Autodesk Fusion 360 part; units mm, degrees
note: some values were not read from the file. Set by a fixed rule: which face or edge a step refers to.
(part 4 of 5)
sketch "Sketch4" plane through (0, 0, 0) normal (1, 0, 0) x (0, 0, -1)
  circle A0 centre (-14.7805, 3.85) radius 2.25 construction
  line L0 (-20.7805, 0) -> (-8.7805, 0) construction
  line L1 (-8.7805, 0) -> (-8.7805, 7.7) construction
  line L2 (-8.7805, 7.7) -> (-20.7805, 7.7) construction
  line L3 (-20.7805, 7.7) -> (-20.7805, 0) construction
  line L4 (8.7805, 0) -> (-8.7805, 0) construction
  line L5 (-8.7805, 0) -> (-8.7805, 7.7) construction
  line L6 (8.7805, 7.7) -> (-8.7805, 7.7) construction
  line L7 (-8.7805, 7.7) -> (-8.7805, 0) construction
  circle A1 centre (-14.7805, 3.85) radius 2.25 construction
  line L8 (-8.7805, 0) -> (-25.7687, 0) construction
  line L9 (-25.7687, 0) -> (-25.7687, 7.7) construction
  line L10 (-25.7687, 7.7) -> (-8.7805, 7.7) construction
  line L11 (-8.7805, 7.7) -> (-8.7805, 0) construction
  line L12 (8.7805, 0) -> (-23.2746, 0)
  line L13 (-23.2746, 0) -> (-23.2746, 7.7)
  line L14 (-23.2746, 7.7) -> (8.7805, 7.7)
  line L15 (8.7805, 7.7) -> (8.7805, 0)
  line L16 (-25.7687, 7.7) -> (-20.7805, 7.7) construction
  line L17 (8.7805, 7.7) -> (8.7805, 0)
  line L18 (8.7805, 0) -> (-8.7805, 0)
  line L19 (8.7805, 0) -> (8.7805, 7.7)
  line L20 (8.7805, 7.7) -> (-8.7805, 7.7)
  circle A2 centre (14.7805, 3.85) radius 2.25
  line L21 (8.7805, 0) -> (20.7805, 0)
  line L22 (20.7805, 0) -> (20.7805, 7.7)
  line L23 (20.7805, 7.7) -> (8.7805, 7.7)
  line L24 (8.7805, 7.7) -> (8.7805, 0)
  constraint horizontal L12
  constraint vertical L13
  constraint horizontal L14
  constraint vertical L15
  constraint coincident L10 L13.end
  constraint coincident L4.start L12.start
  constraint coincident L9.end L10.start
  constraint coincident L2.end L3.start
  constraint midpoint L13.end L16
extrude "Extrude4" cut sketch "Sketch4" against normal blind 9.755
ref_plane "WorkPlane1" through (9.4113, 3.85, 28.5317) normal (-0.487666, 0, 0.87303) x (0.87303, 0, 0.487666)
sketch "Sketch5" plane through (-9.9091, 0, 17.7395) normal (-0.487666, 0, 0.87303) x (0.87303, 0, 0.487666)
  line L0 (7.6399, 0) -> (7.6399, 7.7)
  line L1 (7.6399, 7.7) -> (11.3502, 7.7)
  line L2 (11.3502, 7.7) -> (11.3502, 0)
  line L3 (11.3502, 0) -> (7.6399, 0)
  circle A0 centre (21.8443, 3.85) radius 2.25
  line L4 (35.4044, 0) -> (13.8443, 0)
  line L5 (13.8443, 0) -> (13.8443, 7.7)
  line L6 (13.8443, 7.7) -> (35.4044, 7.7)
  line L7 (35.4044, 7.7) -> (35.4044, 0)
  line L8 (7.6399, 7.7) -> (27.1402, 7.7)
  line L9 (27.1402, 7.7) -> (27.1402, 0)
  line L10 (27.1402, 0) -> (7.6399, 0)
  line L11 (7.6399, 0) -> (7.6399, 7.7)
  line L12 (21.8443, 3.85) -> (21.8443, 7.7) construction
  line L13 (21.8443, 7.7) -> (35.4044, 7.7) construction
  point P0 (27.1402, 8)
  dimension "d37" = 15.79
  constraint horizontal L8
  constraint vertical L9
  constraint horizontal L10
  constraint vertical L11
  constraint coincident L4 L9.end
  constraint coincident L0.end L1.start
  constraint coincident A0.centre L12.start
  constraint coincident L6 L12.end
  constraint vertical L12
  constraint coincident L6.end L7.start
  constraint coincident L9 P0
  measures "d37" distance of L2 L9
extrude "Extrude5" cut sketch "Sketch5" along normal up to surface (4.25 mm away) contours L0 L1 L2 L3 L8 L10 L11 | L2 L5 L8 L10 | L4 L5 L6 L8 L9 L10
sketch "Sketch6" plane through (-11.9817, 0, 21.4499) normal (-0.487666, 0, 0.87303) x (0.87303, 0, 0.487666)
  line L0 (27.1402, 7.7) -> (27.1402, 0)
  line L1 (27.1402, 0) -> (35.4044, 0)
  line L2 (35.4044, 0) -> (35.4044, 7.7)
  line L3 (35.4044, 7.7) -> (27.1402, 7.7)
  line L4 (39.6544, 0) -> (35.4044, 0)
  line L5 (35.4044, 0) -> (35.4044, 7.7)
  line L6 (39.6544, 7.7) -> (35.4044, 7.7)
  line L7 (27.1402, 7.7) -> (39.6544, 7.7)
  line L8 (39.6544, 7.7) -> (39.6544, 0)
  line L9 (39.6544, 0) -> (27.1402, 0)
  line L10 (27.1402, 0) -> (27.1402, 7.7)
  line L11 (35.4044, 7.7) -> (35.4044, 0)
  constraint horizontal L7
  constraint vertical L8
  constraint horizontal L9
  constraint vertical L10
  constraint coincident L4.start L8.end
  constraint coincident L0.start L3.end
extrude "Extrude6" cut sketch "Sketch6" against normal up to surface (8.5 mm away)
equation "d19 = d4"
equation "d20 = ( -d22 / 2 mm ) * 1 mm"
equation "d22 = d1 + 6 mm"
equation "d31 = d32"

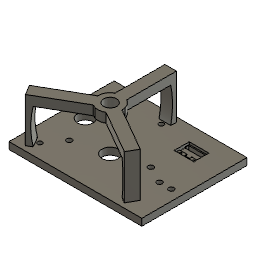
design "Strain Gauge Mount"
Autodesk Fusion 360 part; units mm, degrees
sketch "Sketch1" plane through (0, 0, 0) normal (0, 1, 0) x (1, 0, 0)
  line L0 (-47.5333, 52) -> (47.5333, 52) construction
  line L1 (47.5333, 52) -> (47.5333, -25) construction
  line L2 (47.5333, -25) -> (-47.5333, -25) construction
  line L3 (-47.5333, -25) -> (-47.5333, 52) construction
  line L4 (0, 8) -> (-6.9282, -4) construction
  line L5 (-6.9282, -4) -> (6.9282, -4) construction
  line L6 (6.9282, -4) -> (0, 8) construction
  line L7 (-2.5, 4.3301) -> (2.5, -4.3301) construction
  line L8 (2.5, -4.3301) -> (-42.5333, -30.3301) construction
  line L9 (-42.5333, -30.3301) -> (-47.5333, -21.6699) construction
  line L10 (-47.5333, -21.6699) -> (-2.5, 4.3301) construction
  line L11 (2.5, 4.3301) -> (-2.5, -4.3301) construction
  line L12 (-2.5, -4.3301) -> (42.5333, -30.3301) construction
  line L13 (42.5333, -30.3301) -> (47.5333, -21.6699) construction
  line L14 (2.5, 4.3301) -> (47.5333, -21.6699) construction
  line L15 (-5, 0) -> (-5, 52) construction
  line L16 (-5, 52) -> (5, 52) construction
  line L17 (5, 52) -> (5, 0) construction
  line L18 (5, 0) -> (-5, 0) construction
  line L19 (-5, 52) -> (-5, 2.8868)
  line L20 (-5, 2.8868) -> (-47.5333, -21.6699)
  line L21 (-47.5333, -21.6699) -> (-42.5333, -30.3301)
  line L22 (-42.5333, -30.3301) -> (0, -5.7735)
  line L23 (0, -5.7735) -> (42.5333, -30.3301)
  line L24 (42.5333, -30.3301) -> (47.5333, -21.6699)
  line L25 (47.5333, -21.6699) -> (5, 2.8868)
  line L26 (5, 2.8868) -> (5, 52)
  line L27 (5, 52) -> (-5, 52)
  circle A0 centre (0, 0) radius 10.5
  circle A1 centre (0, 0) radius 7
  dimension "d5" = 60
  dimension "d6" = 60
  dimension "d7" = 4
  dimension "d9" = 4
  dimension "d10" = 4
  dimension "d11" = 10
  dimension "d12" = 5
  dimension "d13" = 5
  dimension "d14" = 10
  dimension "d15" = 10
  dimension "d16" = 5
  dimension "d20" = 52
  dimension "d21" = 52
  dimension "d22" = 52
  dimension "d41" = 21
  dimension "d42" = 14
  constraint horizontal L0
  constraint vertical L1
  constraint horizontal L2
  constraint vertical L3
  constraint perpendicular L3 L5
  constraint parallel L6 L7
  constraint perpendicular L7 L8
  constraint coincident L3 L9.end
  constraint perpendicular L8 L9
  constraint perpendicular L7 L10
  constraint coincident A0.centre L7
  constraint perpendicular L11 L12
  constraint coincident L1 L13.end
  constraint perpendicular L12 L13
  constraint coincident A0.centre L11
  constraint perpendicular L13 L14
  constraint parallel L4 L11
  constraint coincident L0 L15.end
  constraint perpendicular L0 L15
  constraint coincident L0 L16.end
  constraint perpendicular L16 L17
  constraint perpendicular L17 L18
  constraint coincident A0.centre L18
  constraint coincident L15 L19.end
  constraint coincident L10 L19.end
  constraint perpendicular L9 L20
  constraint perpendicular L8 L21
  constraint coincident L12 L22.end
  constraint coincident L8 L22.end
  constraint coincident L17 L25.end
  constraint coincident L14 L25.end
  constraint coincident A0.centre A1.centre
  measures "d5" angle of L4 L5
  measures "d6" angle of L5 L6
  measures "d7" distance of A0.centre L5
  measures "d9" distance of A0.centre L6
  measures "d10" distance of A0.centre L4
  measures "d11" distance of L8.end L9.end
  measures "d12" distance of A0.centre L10
  measures "d13" distance of A0.centre L11.start
  measures "d14" distance of L12.end L13.end
  measures "d15" distance of L15 L17
  measures "d16" distance of A0.centre L15
  measures "d20" distance of L7.start L9.end
  measures "d21" distance of L11.start L13.end
  measures "d22" distance of L15.start L15.end
  measures "d41" diameter of A0
  measures "d42" diameter of A1
extrude "Extrude1" add sketch "Sketch1" along normal blind 6
sketch "Sketch2" plane through (0, 6, 0) normal (0, 1, 0) x (-1, 0, 0)
  line L0 (-5, -52) -> (5, -52)
  line L1 (5, -52) -> (5, -9.2331)
  line L2 (10.4961, 0.2864) -> (47.5333, 21.6699)
  line L3 (47.5333, 21.6699) -> (42.5333, 30.3301)
  line L4 (42.5333, 30.3301) -> (5.4961, 8.9467)
  line L5 (-5.4961, 8.9467) -> (-42.5333, 30.3301)
  line L6 (-42.5333, 30.3301) -> (-47.5333, 21.6699)
  line L7 (-47.5333, 21.6699) -> (-10.4961, 0.2864)
  line L8 (-5, -9.2331) -> (-5, -52)
  line L9 (5, -52) -> (-5, -52)
  line L10 (-5, -52) -> (-5, -47)
  line L11 (-5, -47) -> (5, -47)
  line L12 (5, -47) -> (5, -52)
  line L13 (43.2032, 19.1699) -> (38.2032, 27.8301)
  line L14 (43.2032, 19.1699) -> (47.5333, 21.6699)
  line L15 (47.5333, 21.6699) -> (42.5333, 30.3301)
  line L16 (42.5333, 30.3301) -> (38.2032, 27.8301)
  line L17 (-47.5333, 21.6699) -> (-42.5333, 30.3301)
  line L18 (-42.5333, 30.3301) -> (-38.2032, 27.8301)
  line L19 (-38.2032, 27.8301) -> (-43.2032, 19.1699)
  line L20 (-43.2032, 19.1699) -> (-47.5333, 21.6699)
  arc A0 (-10.4961, 0.2864) -> (-5, -9.2331) centre (0, 0) ccw
  arc A1 (5, -9.2331) -> (10.4961, 0.2864) centre (0, 0) ccw
  arc A2 (5.4961, 8.9467) -> (-5.4961, 8.9467) centre (0, 0) ccw
  dimension "d25" = 5
  dimension "d26" = 5
  dimension "d27" = 5
  constraint horizontal L9
  constraint vertical L10
  constraint horizontal L11
  constraint vertical L12
  constraint coincident L8 L10.end
  constraint coincident L0.end L1.start
  constraint coincident L2 L13.start
  constraint coincident L4 L13.end
  constraint perpendicular L4 L13
  constraint coincident L2.end L3.start
  constraint coincident L3.end L4.start
  constraint coincident L6.end L7.start
  constraint coincident L5.end L6.start
  constraint coincident L5 L18.end
  constraint coincident L7 L19.end
  constraint perpendicular L7 L19
  measures "d25" distance of L0.start L10.end
  measures "d26" distance of L13.start L2.end
  measures "d27" distance of L6.end L19.end
extrude "Extrude2" add sketch "Sketch2" along normal blind 30 contours L0 L1 L8 L9 L10 L11 L12 | L5 L6 L7 L17 L18 L19 L20 | L2 L3 L4 L13 L14 L15 L16
sketch "Sketch3" plane through (0, 36, 0) normal (0, 1, 0) x (-1, 0, 0)
  line L0 (43.2032, 19.1699) -> (47.5333, 21.6699)
  line L1 (47.5333, 21.6699) -> (42.5333, 30.3301)
  line L2 (42.5333, 30.3301) -> (38.2032, 27.8301)
  line L3 (38.2032, 27.8301) -> (43.2032, 19.1699)
  line L4 (-38.2032, 27.8301) -> (-43.2032, 19.1699)
  line L5 (-43.2032, 19.1699) -> (-10.4961, 0.2864)
  line L6 (-5, -9.2331) -> (-5, -47)
  line L7 (-5, -47) -> (5, -47)
  line L8 (5, -47) -> (5, -9.2331)
  line L9 (10.4961, 0.2864) -> (43.2032, 19.1699)
  line L10 (43.2032, 19.1699) -> (38.2032, 27.8301)
  line L11 (38.2032, 27.8301) -> (5.4961, 8.9467)
  line L12 (-5.4961, 8.9467) -> (-38.2032, 27.8301)
  line L13 (5, -47) -> (-5, -47)
  line L14 (-5, -47) -> (-5, -52)
  line L15 (-5, -52) -> (5, -52)
  line L16 (5, -52) -> (5, -47)
  line L17 (-43.2032, 19.1699) -> (-38.2032, 27.8301)
  line L18 (-38.2032, 27.8301) -> (-42.5333, 30.3301)
  line L19 (-42.5333, 30.3301) -> (-47.5333, 21.6699)
  line L20 (-47.5333, 21.6699) -> (-43.2032, 19.1699)
  line L21 (47.5333, 21.6699) -> (5, -9.2331)
  line L22 (5, -9.2331) -> (5, -52)
  line L23 (5, -52) -> (-5, -52)
  line L24 (-5, -52) -> (-10.4961, 0.2864)
  line L25 (-10.4961, 0.2864) -> (-47.5333, 21.6699)
  line L26 (-47.5333, 21.6699) -> (-42.5333, 30.3301)
  line L27 (-42.5333, 30.3301) -> (5.4961, 8.9467)
  line L28 (5.4961, 8.9467) -> (42.5333, 30.3301)
  line L29 (42.5333, 30.3301) -> (47.5333, 21.6699)
  line L30 (5, -9.5295) -> (-9.3062, -11.0333) construction
  line L31 (-10.7528, 0.4346) -> (-6.6754, 9.5928) construction
  line L32 (13.3677, -3.1535) -> (6.1603, 9.3301) construction
  circle A0 centre (0, 0) radius 10
  circle A1 centre (0, 0) radius 5.375
  arc A2 (-10.4961, 0.2864) -> (-5, -9.2331) centre (0, 0) ccw
  arc A3 (5, -9.2331) -> (10.4961, 0.2864) centre (0, 0) ccw
  arc A4 (5.4961, 8.9467) -> (-5.4961, 8.9467) centre (0, 0) ccw
  dimension "d33" = 10
  dimension "d34" = 10
  dimension "d35" = 10
  dimension "d40" = 10.75
  constraint coincident L0.end L1.start
  constraint coincident L8.end L21.end
  constraint coincident L15.end L16.start
  constraint coincident L14.end L15.start
  constraint coincident L5.end L24.end
  constraint coincident L19.end L20.start
  constraint coincident L18.end L19.start
  constraint coincident L11.end L27.end
  constraint coincident L1.end L2.start
  constraint coincident L8 L30.start
  constraint coincident L24 L30.end
  constraint perpendicular L24 L30
  constraint coincident L25 L31.start
  constraint perpendicular L27 L31
  constraint coincident L21 L32.start
  constraint coincident L11 L32.end
  constraint perpendicular L28 L32
  constraint concentric A0 A1
  measures "d33" distance of A0.centre L32
  measures "d34" distance of A0.centre L30
  measures "d35" distance of A0.centre L31
  measures "d40" diameter of A1
extrude "Extrude3" add sketch "Sketch3" along normal blind 8 contours L0 L1 L2 L3 L10 L28 L29 | L3 L4 L5 L6 L7 L8 L9 L10 L11 L12 L13 L17 L21 L22 L24 L25 L27 L28 A2 A3 A4 | L7 L13 L14 L15 L16 L22 L23 | L4 L17 L18 L19 L20 L25 L26 | A0 | A1
sketch "Sketch5" plane through (0, 44, 0) normal (0, 1, 0) x (-1, 0, 0)
  line L0 (40.8013, 29.3301) -> (5, 8.6603)
  arc A0 (5, 8.6603) -> (-5, 8.6603) centre (0, 0) ccw
  line L1 (-5, 8.6603) -> (-40.8013, 29.3301)
  line L2 (-40.8013, 29.3301) -> (-45.8013, 20.6699)
  line L3 (-45.8013, 20.6699) -> (-10, 0)
  arc A1 (-10, 0) -> (-5, -8.6603) centre (0, 0) ccw
  line L4 (-5, -8.6603) -> (-5, -50)
  line L5 (-5, -50) -> (5, -50)
  line L6 (5, -50) -> (5, -8.6603)
  arc A2 (5, -8.6603) -> (10, 0) centre (0, 0) ccw
  line L7 (10, 0) -> (45.8013, 20.6699)
  line L8 (45.8013, 20.6699) -> (40.8013, 29.3301)
  circle A3 centre (0, 0) radius 5.6417
  line L9 (-5.4961, 8.9467) -> (-42.5333, 30.3301)
  line L10 (-42.5333, 30.3301) -> (-47.5333, 21.6699)
  line L11 (-47.5333, 21.6699) -> (-10.4961, 0.2864)
  line L12 (-5, -9.2331) -> (-5, -52)
  line L13 (-5, -52) -> (5, -52)
  line L14 (5, -52) -> (5, -9.2331)
  line L15 (5, -9.2331) -> (7.2363, -7.6083)
  line L16 (47.5333, 21.6699) -> (42.5333, 30.3301)
  line L17 (42.5333, 30.3301) -> (5.4961, 8.9467)
  line L18 (-10.4961, 0.2864) -> (-10.2071, -2.4626)
  line L19 (5.4961, 8.9467) -> (2.9709, 10.0709)
  arc A4 (2.9709, 10.0709) -> (-5.4961, 8.9467) centre (0, 0) ccw
  arc A5 (-10.2071, -2.4626) -> (-5, -9.2331) centre (0, 0) ccw
  arc A6 (7.2363, -7.6083) -> (10.4961, 0.2864) centre (0, 0) ccw
  line L20 (10.4961, 0.2864) -> (47.5333, 21.6699)
  dimension "d39" = 11.2833
  constraint concentric A0 A3
  measures "d39" diameter of A3
loft "Loft1" cut profiles "Sketch5", "Sketch3" section 1 contours A3 section 2 contours A1
sketch "Sketch6" plane through (0, 6, 0) normal (0, 1, 0) x (-1, 0, 0)
  line L0 (-38.2032, 27.8301) -> (-43.2032, 19.1699)
  line L1 (-43.2032, 19.1699) -> (-10.4961, 0.2864)
  arc A0 (-10.4961, 0.2864) -> (-5, -9.2331) centre (0, 0) ccw
  line L2 (-5, -9.2331) -> (-5, -47)
  line L3 (-5, -47) -> (5, -47)
  line L4 (5, -47) -> (5, -9.2331)
  arc A1 (5, -9.2331) -> (10.4961, 0.2864) centre (0, 0) ccw
  line L5 (10.4961, 0.2864) -> (43.2032, 19.1699)
  line L6 (43.2032, 19.1699) -> (38.2032, 27.8301)
  line L7 (38.2032, 27.8301) -> (5.4961, 8.9467)
  arc A2 (5.4961, 8.9467) -> (-5.4961, 8.9467) centre (0, 0) ccw
  line L8 (-5.4961, 8.9467) -> (-38.2032, 27.8301)
  circle A3 centre (0, 0) radius 7
  dimension "d43" = 14
  constraint coincident A0.centre A1.centre
  measures "d43" diameter of A3
loft "Loft2" cut profiles "Sketch1", "Sketch6" section 1 contours L19 L20 L22 L23 L25 L26 A1 | L19 L20 A1 | L25 L26 A1 | L22 L23 A1 section 2 contours A3
sketch "Sketch9" plane through (2.5, 0, 4.3301) normal (0.5, 0, 0.866025) x (0.866025, 0, -0.5)
  line L0 (-9.2331, 6) -> (-47, 6)
  line L1 (-47, 6) -> (-47, 36)
  line L2 (-47, 36) -> (-9.2331, 36)
  line L3 (-9.2331, 36) -> (-9.2331, 44)
  line L4 (-9.2331, 44) -> (-52, 44)
  line L5 (-52, 44) -> (-52, 0)
  arc A0 (-47, 36) -> (-47, 6) centre (26.4847, 21) ccw
  line L6 (-47, 21) -> (81, 21) construction
  line L7 (-52, 0) -> (-9.2331, 0)
  line L8 (-9.2331, 0) -> (-9.2331, 6)
  dimension "d61" = 75
  constraint coincident L0.end L1.start
  constraint coincident L1.end L2.start
  constraint coincident L1 L6.start
  constraint perpendicular L1 L6
  constraint midpoint L1 L6.start
  measures "d61" radius of A0
extrude "Extrude7" cut sketch "Sketch9" against normal up to surface (10 mm away) contours L1 A0
sketch "Sketch10" plane through (-2.5, 0, 4.3301) normal (-0.5, 0, 0.866025) x (0.866025, 0, 0.5)
  line L0 (47, 6) -> (9.2331, 6)
  line L1 (52, 0) -> (52, 44)
  line L2 (52, 44) -> (9.2331, 44)
  line L3 (9.2331, 36) -> (47, 36)
  line L4 (47, 36) -> (47, 6)
  arc A0 (47, 6) -> (47, 36) centre (-26.4847, 21) ccw
  line L5 (9.2331, 0) -> (52, 0)
  line L6 (9.2331, 6) -> (9.2331, 0)
  line L7 (9.2331, 44) -> (9.2331, 36)
  dimension "d64" = 75
  constraint coincident L0.start L4.end
  constraint coincident L3.end L4.start
  measures "d64" radius of A0
extrude "Extrude8" cut sketch "Sketch10" against normal up to surface (10 mm away) contours L4 A0
sketch "Sketch11" plane through (5, 0, 0) normal (1, 0, 0) x (0, 0, -1)
  line L0 (47, 6) -> (9.2331, 6)
  line L1 (52, 0) -> (52, 44)
  line L2 (52, 44) -> (9.2331, 44)
  line L3 (47, 36) -> (47, 6)
  arc A0 (47, 6) -> (47, 36) centre (-26.4847, 21) ccw
  line L4 (9.2331, 36) -> (47, 36)
  line L5 (9.2331, 0) -> (52, 0)
  line L6 (9.2331, 6) -> (9.2331, 0)
  line L7 (9.2331, 44) -> (9.2331, 36)
  dimension "d67" = 75
  constraint coincident L0.start L3.end
  constraint coincident L3.start A0.end
  measures "d67" radius of A0
extrude "Extrude9" cut sketch "Sketch11" against normal up to surface (10 mm away) contours L3 A0
sketch "Sketch7" plane through (0, 6, 0) normal (0, 1, 0) x (-1, 0, 0)
  circle A0 centre (0, 0) radius 7
  line L0 (-43.2032, 19.1699) -> (-10.4961, 0.2864)
  arc A1 (-10.4961, 0.2864) -> (-5, -9.2331) centre (0, 0) ccw
  line L1 (-5, -9.2331) -> (-5, -47)
  line L2 (5, -47) -> (5, -9.2331)
  arc A2 (5, -9.2331) -> (10.4961, 0.2864) centre (0, 0) ccw
  line L3 (10.4961, 0.2864) -> (43.2032, 19.1699)
  line L4 (38.2032, 27.8301) -> (5.4961, 8.9467)
  arc A3 (5.4961, 8.9467) -> (-5.4961, 8.9467) centre (0, 0) ccw
  line L5 (-5.4961, 8.9467) -> (-38.2032, 27.8301)
  line L6 (52.5333, -56) -> (-61.5333, -56)
  line L7 (-61.5333, -56) -> (-61.5333, 34.3301)
  line L8 (-61.5333, 34.3301) -> (52.5333, 34.3301)
  line L9 (52.5333, 34.3301) -> (52.5333, -56)
  line L10 (47.5333, 21.6699) -> (42.5333, 30.3301)
  line L11 (-42.5333, 30.3301) -> (-47.5333, 21.6699)
  line L12 (-5, -52) -> (5, -52) construction
  line L13 (-38.2032, 27.8301) -> (-43.2032, 19.1699)
  line L14 (-5, -47) -> (5, -47)
  line L15 (43.2032, 19.1699) -> (38.2032, 27.8301)
  dimension "d51" = 4
  dimension "d139" = 5
  dimension "d141" = 14
  dimension "d142" = 4
  constraint horizontal L6
  constraint vertical L7
  constraint horizontal L8
  constraint vertical L9
  measures "d51" distance of L6 L12
  measures "d139" distance of L9 L10.start
  measures "d141" distance of L7 L11.end
  measures "d142" distance of L8 L10.end
extrude "Extrude5" add sketch "Sketch7" against normal blind 6 contours L6 L7 L8 L9
sketch "Sketch14" plane through (0, 0, 0) normal (0, -1, 0) x (1, 0, 0)
  line L0 (61.5333, 34.3301) -> (-52.5333, 34.3301)
  line L1 (-52.5333, 34.3301) -> (-52.5333, -56)
  line L2 (-52.5333, -56) -> (61.5333, -56)
  line L3 (61.5333, -56) -> (61.5333, 34.3301)
  circle A0 centre (27.456, -7.5) radius 2.25
  circle A1 centre (-27.456, 7.5) radius 2.25
  circle A2 centre (27.456, 7.5) radius 2.25
  line L4 (0, 0) -> (61.5333, 0) construction
  circle A3 centre (42.456, 0) radius 2.25
  circle A4 centre (52.456, 0) radius 2.25
  circle A5 centre (0, 0) radius 7
  dimension "d86" = 27.456
  dimension "d88" = 27.456
  dimension "d89" = 27.456
  dimension "d90" = 7.5
  dimension "d92" = 7.5
  dimension "d93" = 7.5
  dimension "d94" = 4.5
  dimension "d96" = 4.5
  dimension "d97" = 4.5
  dimension "d100" = 4.5
  dimension "d101" = 15
  dimension "d102" = 4.5
  dimension "d103" = 10
  dimension "d104" = 19.0773
  constraint coincident L3 L4.end
  constraint perpendicular L3 L4
  constraint coincident L4 A3.centre
  constraint coincident L4 A4.centre
  measures "d86" horizontal distance of L4.start A0.centre
  measures "d88" horizontal distance of L4.start A2.centre
  measures "d89" horizontal distance of L4.start A1.centre
  measures "d90" vertical distance of L4.start A0.centre
  measures "d92" vertical distance of L4.start A2.centre
  measures "d93" vertical distance of L4.start A1.centre
  measures "d94" diameter of A0
  measures "d96" diameter of A2
  measures "d97" diameter of A1
  measures "d100" diameter of A3
  measures "d101" horizontal distance of A0.centre A3.centre
  measures "d102" diameter of A4
  measures "d103" distance of A3.centre A4.centre
  measures "d104" distance of L3 A3.centre
extrude "Extrude12" cut sketch "Sketch14" against normal blind 8 contours A0 | A1 | A2 | A3 | A4
sketch "Sketch15" plane through (0, 6, 0) normal (0, 1, 0) x (-1, 0, 0)
  circle A0 centre (27.456, 7.5) radius 2.25
  circle A1 centre (-27.456, -7.5) radius 2.25
  circle A2 centre (-42.456, 0) radius 2.25
  circle A3 centre (-27.456, 7.5) radius 2.25
  circle A4 centre (-52.456, 0) radius 2.25
  line L0 (-5, -47) -> (5, -47)
  line L1 (5, -47) -> (5, -52)
  line L2 (5, -52) -> (-5, -52)
  line L3 (-5, -52) -> (-5, -47)
  line L4 (43.2032, 19.1699) -> (38.2032, 27.8301)
  line L5 (38.2032, 27.8301) -> (42.5333, 30.3301)
  line L6 (42.5333, 30.3301) -> (47.5333, 21.6699)
  line L7 (47.5333, 21.6699) -> (43.2032, 19.1699)
  line L8 (52.5333, 34.3301) -> (-61.5333, 34.3301)
  line L9 (-61.5333, 34.3301) -> (-61.5333, -56)
  line L10 (-61.5333, -56) -> (52.5333, -56)
  line L11 (52.5333, -56) -> (52.5333, 34.3301)
  circle A5 centre (0, 0) radius 7
  line L12 (-43.2032, 19.1699) -> (-47.5333, 21.6699)
  line L13 (-47.5333, 21.6699) -> (-42.5333, 30.3301)
  line L14 (-42.5333, 30.3301) -> (-38.2032, 27.8301)
  line L15 (-38.2032, 27.8301) -> (-43.2032, 19.1699)
  line L16 (-39.097, -32.667) -> (-25, -32.667) construction
  line L17 (-26.692, -32.667) -> (-26.692, -42.8778) construction
  circle A6 centre (-27.667, -32.667) radius 0.975
  line L18 (-27.667, -32.667) -> (-41.764, -32.667) construction
  line L19 (-25, -30) -> (-25, -42.8778)
  line L20 (-40.072, -32.667) -> (-40.072, -42.8778) construction
  line L21 (-41.764, -30) -> (-25, -30)
  circle A7 centre (-39.097, -32.667) radius 0.975
  line L22 (-41.764, -42.8778) -> (-41.764, -30)
  line L23 (-25, -42.8778) -> (-41.764, -42.8778)
  line L24 (-26.692, -39.1346) -> (-25, -39.1346) construction
  line L25 (-26.692, -39.1346) -> (-41.764, -39.1346) construction
  line L26 (-41.764, -39.1346) -> (-41.764, -34.6346)
  line L27 (-41.764, -34.6346) -> (-25, -34.6346)
  line L28 (-25, -34.6346) -> (-25, -39.1346)
  line L29 (-31.267, -34.6346) -> (-35.497, -34.6346)
  line L30 (-35.497, -34.6346) -> (-35.497, -32.6346)
  line L31 (-35.497, -32.6346) -> (-31.267, -32.6346)
  line L32 (-31.267, -32.6346) -> (-31.267, -34.6346)
  line L33 (-25.492, -41.8778) -> (-41.272, -41.8778)
  line L34 (-41.272, -41.8778) -> (-41.272, -39.1346)
  line L35 (-41.272, -39.1346) -> (-25.492, -39.1346)
  line L36 (-25.492, -39.1346) -> (-25.492, -41.8778)
  line L37 (-25.492, -39.1346) -> (-25, -39.1346)
  line L38 (-41.272, -39.1346) -> (-41.764, -39.1346)
  dimension "d105" = 12.8778
  dimension "d106" = 16.764
  dimension "d107" = 2.667
  dimension "d108" = 2.667
  dimension "d109" = 2.667
  dimension "d110" = 2.667
  dimension "d111" = 1.95
  dimension "d112" = 1.95
  dimension "d117" = 4.5
  dimension "d118" = 6.5
  dimension "d119" = 3.6
  dimension "d120" = 3.6
  dimension "d121" = 3.7432
  dimension "d122" = 1
  dimension "d123" = 1.2
  dimension "d124" = 1.2
  dimension "d143" = 30
  dimension "d144" = 25
  constraint coincident L16.start A7.centre
  constraint coincident L16.end L19
  constraint perpendicular L16 L19
  constraint coincident A6.centre L18.start
  constraint coincident L18.end L22
  constraint perpendicular L18 L22
  constraint coincident L20.start A7
  constraint coincident L20.start L18
  constraint coincident L20.end L23
  constraint tangent L20 A7
  constraint coincident L17.start L16
  constraint coincident L17.start A6
  constraint coincident L17.end L23
  constraint tangent L17 A6
  constraint coincident L24.start L17
  constraint perpendicular L19 L23
  constraint perpendicular L19 L21
  constraint perpendicular L21 L22
  constraint horizontal L23
  constraint coincident L19 L24.end
  constraint perpendicular L19 L24
  constraint coincident L22 L25.end
  constraint perpendicular L22 L25
  constraint vertical L26
  constraint horizontal L27
  constraint vertical L28
  constraint coincident L22 L26.end
  constraint horizontal L29
  constraint vertical L30
  constraint horizontal L31
  constraint vertical L32
  constraint coincident L27 L29.start
  constraint horizontal L33
  constraint vertical L34
  constraint horizontal L35
  constraint vertical L36
  constraint coincident L25 L34.end
  constraint perpendicular L22 L38
  measures "d105" distance of L22.start L21.start
  measures "d106" distance of L21.start L19.start
  measures "d107" distance of A6.centre L21
  measures "d108" distance of L16.start L21
  measures "d109" distance of L16.start L22
  measures "d110" distance of A6.centre L19
  measures "d111" diameter of A7
  measures "d112" diameter of A6
  measures "d117" distance of L25 L27
  measures "d118" distance of L25 L31
  measures "d119" distance of A6.centre L32
  measures "d120" distance of L16.start L30
  measures "d121" distance of L23 L25
  measures "d122" distance of L23 L33
  measures "d123" distance of L17 L36
  measures "d124" distance of L20 L34
  measures "d143" distance of A5.centre L21
  measures "d144" distance of A5.centre L19
extrude "Extrude13" cut sketch "Sketch15" against normal up to surface (6 mm away) contours A6 | L33 L34 L35 L36 | A7
extrude "Extrude14" cut sketch "Sketch15" against normal blind 2.7 contours L19 L22 L26 L27 L28 L29 L35 L37 L38 | L27 L29 L30 L31 L32
extrude "Extrude15" cut sketch "Sketch15" against normal blind 2 contours L19 L21 L22 L27 L30 L31 L32 | L19 L22 L23 L33 L34 L36 L37 L38
sketch "Sketch16" plane through (0, 6, 0) normal (0, 1, 0) x (-1, 0, 0)
  line L0 (-25, -30) -> (-25, -42.8778)
  line L1 (-25, -42.8778) -> (-41.764, -42.8778)
  line L2 (-41.764, -42.8778) -> (-41.764, -30)
  line L3 (-41.764, -30) -> (-25, -30)
  circle A0 centre (27.456, 7.5) radius 2.25
  circle A1 centre (-27.456, -7.5) radius 2.25
  circle A2 centre (-42.456, 0) radius 2.25
  circle A3 centre (-27.456, 7.5) radius 2.25
  circle A4 centre (-52.456, 0) radius 2.25
  line L4 (-5, -47) -> (5, -47)
  line L5 (5, -47) -> (5, -52)
  line L6 (5, -52) -> (-5, -52)
  line L7 (-5, -52) -> (-5, -47)
  line L8 (43.2032, 19.1699) -> (38.2032, 27.8301)
  line L9 (38.2032, 27.8301) -> (42.5333, 30.3301)
  line L10 (42.5333, 30.3301) -> (47.5333, 21.6699)
  line L11 (47.5333, 21.6699) -> (43.2032, 19.1699)
  line L12 (52.5333, 34.3301) -> (-61.5333, 34.3301)
  line L13 (-61.5333, 34.3301) -> (-61.5333, -56)
  line L14 (-61.5333, -56) -> (52.5333, -56)
  line L15 (52.5333, -56) -> (52.5333, 34.3301)
  circle A5 centre (0, 0) radius 7
  line L16 (-43.2032, 19.1699) -> (-47.5333, 21.6699)
  line L17 (-47.5333, 21.6699) -> (-42.5333, 30.3301)
  line L18 (-42.5333, 30.3301) -> (-38.2032, 27.8301)
  line L19 (-38.2032, 27.8301) -> (-43.2032, 19.1699)
  circle A6 centre (36.9738, -15.59) radius 6.75
  line L20 (36.9738, -15.59) -> (43.7238, -15.59) construction
  line L21 (36.9738, -15.59) -> (36.9738, -22.34) construction
  dimension "d132" = 13.5
  dimension "d145" = 36.9738
  dimension "d146" = 15.59
  dimension "d147" = 8.8095
  dimension "d148" = 33.66
  constraint coincident A6.centre L20.start
  constraint coincident A6 L20.end
  constraint horizontal L20
  constraint coincident A6 L21.end
  constraint perpendicular L20 L21
  measures "d132" diameter of A6
  measures "d145" horizontal distance of A5.centre A6.centre
  measures "d146" vertical distance of A5.centre A6.centre
  measures "d147" distance of L15 L20.end
  measures "d148" distance of L14 L21.end
extrude "Extrude16" cut sketch "Sketch16" against normal up to surface (6 mm away) contours A6
sketch "Sketch17" plane through (0, 6, 0) normal (0, 1, 0) x (-1, 0, 0)
  circle A0 centre (36.9738, -15.59) radius 6.75
  line L0 (-25, -30) -> (-25, -42.8778)
  line L1 (-25, -42.8778) -> (-41.764, -42.8778)
  line L2 (-41.764, -42.8778) -> (-41.764, -30)
  line L3 (-41.764, -30) -> (-25, -30)
  circle A1 centre (27.456, 7.5) radius 2.25
  circle A2 centre (-27.456, 7.5) radius 2.25
  circle A3 centre (-42.456, 0) radius 2.25
  circle A4 centre (-27.456, -7.5) radius 2.25
  circle A5 centre (-52.456, 0) radius 2.25
  line L4 (-5, -47) -> (5, -47)
  line L5 (5, -47) -> (5, -52)
  line L6 (5, -52) -> (-5, -52)
  line L7 (-5, -52) -> (-5, -47)
  line L8 (-43.2032, 19.1699) -> (-47.5333, 21.6699)
  line L9 (-47.5333, 21.6699) -> (-42.5333, 30.3301)
  line L10 (-42.5333, 30.3301) -> (-38.2032, 27.8301)
  line L11 (-38.2032, 27.8301) -> (-43.2032, 19.1699)
  line L12 (52.5333, 34.3301) -> (-61.5333, 34.3301)
  line L13 (-61.5333, 34.3301) -> (-61.5333, -56)
  line L14 (-61.5333, -56) -> (52.5333, -56)
  line L15 (52.5333, -56) -> (52.5333, 34.3301)
  circle A6 centre (0, 0) radius 7
  line L16 (38.2032, 27.8301) -> (42.5333, 30.3301)
  line L17 (42.5333, 30.3301) -> (47.5333, 21.6699)
  line L18 (47.5333, 21.6699) -> (43.2032, 19.1699)
  line L19 (43.2032, 19.1699) -> (38.2032, 27.8301)
  line L20 (-38.2032, 27.8301) -> (-43.2032, 19.1699)
  line L21 (43.2032, 19.1699) -> (38.2032, 27.8301)
  line L22 (-5, -47) -> (5, -47)
  line L23 (40.7032, 23.5) -> (0, 0) construction
  line L24 (0, 0) -> (-40.7032, 23.5) construction
  line L25 (0, 0) -> (0, -47) construction
  circle A7 centre (38.1051, 22) radius 2
  circle A8 centre (-38.1051, 22) radius 2
  circle A9 centre (0, -44) radius 2
  point P0 (39.8372, 23)
  point P1 (-39.8372, 23)
  point P2 (0, -46)
  dimension "d149" = 4
  dimension "d150" = 4
  dimension "d151" = 4
  dimension "d152" = 1
  dimension "d153" = 1
  dimension "d154" = 1
  constraint midpoint L19 L23.start
  constraint coincident A6.centre L23.end
  constraint midpoint L11 L24.end
  constraint midpoint L4 L25.end
  constraint coincident L23 A7.centre
  constraint coincident L24 A8.centre
  constraint coincident L25 A9.centre
  constraint coincident A7 P0
  constraint coincident L23 P0
  constraint coincident L24 P1
  constraint coincident A8 P1
  constraint coincident A9 P2
  constraint coincident L25 P2
  measures "d149" diameter of A7
  measures "d150" diameter of A9
  measures "d151" diameter of A8
  measures "d152" distance of L23.start P0
  measures "d153" distance of L25.end P2
  measures "d154" distance of L24.end P1
extrude "Extrude17" cut sketch "Sketch17" against normal up to surface (6 mm away) contours A7 | A8 | A9
equation "d6 = d5"
equation "d9 = d7"
equation "d10 = d7"
equation "d12 = d11 / 2"
equation "d13 = d14 / 2"
equation "d14 = d11"
equation "d15 = d11"
equation "d16 = d15 / 2"
equation "d21 = d20"
equation "d22 = d20"
equation "d23 = 6.00 mm"
equation "d26 = d25"
equation "d27 = d25"
equation "d34 = d33"
equation "d35 = d33"
equation "d39 = d40 + ( 8 / 15 ) * 1 mm"
equation "d53 = -d23"
equation "d64 = d61"
equation "d67 = d61"
equation "d88 = d86"
equation "d89 = d86"
equation "d92 = d90"
equation "d93 = d90"
equation "d96 = d94"
equation "d97 = d94"
equation "d100 = d94"
equation "d102 = d94"
equation "d108 = d107"
equation "d109 = d107"
equation "d110 = d107"
equation "d112 = d111"
equation "d120 = d119"
equation "d124 = d123"
equation "d142 = d51"
equation "d150 = d149"
equation "d151 = d149"
equation "d153 = d152"
equation "d154 = d152"

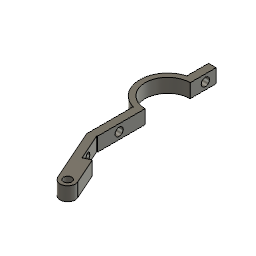
design "Trumpet Clamp 3 Main"
Autodesk Fusion 360 part; units mm, degrees
sketch "Sketch1" plane through (0, 0, 0) normal (0, 1, 0) x (1, 0, 0)
  circle A0 centre (0, 0) radius 12.435
  circle A1 centre (0, 0) radius 15.435
  line L0 (0, 0) -> (-15.435, 0) construction
  line L1 (0, 0) -> (15.435, 0) construction
  line L2 (-4.25, -40.647) -> (8.6182, -69.5153)
  line L3 (4.25, -38.8384) -> (16.3818, -66.0547)
  circle A2 centre (12.5, -67.785) radius 4.25
  line L4 (12.5, -67.785) -> (8.6182, -69.5153) construction
  line L5 (12.5, -67.785) -> (16.3818, -66.0547) construction
  circle A3 centre (12.5, -67.785) radius 2.25
  line L6 (-4.25, -40.647) -> (-4.25, -14.8384)
  line L7 (4.25, -38.8384) -> (4.25, -14.8384)
  line L8 (0, 0) -> (0, -38.8384) construction
  line L9 (4.25, -38.8384) -> (-4.25, -38.8384) construction
  line L10 (-4.25, 14.8384) -> (-4.25, 26.8384)
  line L11 (-4.25, 26.8384) -> (4.25, 26.8384)
  line L12 (4.25, 26.8384) -> (4.25, 14.8384)
  line L13 (-4.25, 14.8384) -> (-4.25, -14.8384) construction
  line L14 (4.25, -14.8384) -> (4.25, 14.8384) construction
  line L15 (12.5, -67.785) -> (12.5, -72.035) construction
  point P0 (0, -15.435)
  dimension "d1" = 24.87
  dimension "d3" = 4.5
  dimension "d4" = 8.5
  dimension "d5" = 12.5
  dimension "d19" = 8.5
  dimension "d22" = 30.87
  dimension "d27" = 24
  dimension "d28" = 12
  dimension "d32" = 56.6
  constraint coincident A0.centre A1.centre
  constraint concentric A0 A1
  constraint coincident A1 L0.end
  constraint horizontal L0
  constraint coincident A1 L1.end
  constraint parallel L0 L1
  constraint coincident A2.centre L4.start
  constraint coincident A2 L2.end
  constraint coincident A2 L3.end
  constraint parallel L4 L5
  constraint coincident L2.end L4.end
  constraint coincident L3.end L5.end
  constraint coincident A1 L6.end
  constraint coincident A1 L7.end
  constraint parallel L2 L3
  constraint vertical L6
  constraint vertical L7
  constraint vertical L8
  constraint tangent L3 A2
  constraint coincident L6 L9.end
  constraint perpendicular L6 L9
  constraint midpoint L8.end L9
  constraint coincident A1 L10.start
  constraint vertical L10
  constraint perpendicular L10 L11
  constraint coincident A1 L12.end
  constraint perpendicular L11 L12
  constraint vertical L13
  constraint vertical L14
  constraint coincident A2 L15.end
  constraint vertical L15
  constraint coincident A1 P0
  constraint coincident L8 P0
  measures "d1" diameter of A0
  measures "d3" diameter of A3
  measures "d4" diameter of A2
  measures "d5" horizontal distance of A0.centre A2.centre
  measures "d19" distance of L6 L7
  measures "d22" diameter of A1
  measures "d27" distance of L3.start L7.end
  measures "d28" distance of L11.end L12.end
  measures "d32" vertical distance of L15.end P0
extrude "Extrude1" add sketch "Sketch1" along normal blind 7.7
sketch "Sketch2" plane through (-10.8972, 0, 4.8575) normal (0.913367, 0, -0.407138) x (-0.407138, 0, -0.913367)
  line L0 (-67.0018, 0) -> (-37.204, 0)
  line L1 (-37.204, 0) -> (-37.204, 7.7)
  line L2 (-37.204, 7.7) -> (-67.0018, 7.7)
  line L3 (-67.0018, 7.7) -> (-67.0018, 0)
  line L4 (-37.204, 3.85) -> (-67.0018, 3.85) construction
  circle A0 centre (-45.204, 3.85) radius 2.25
  dimension "d29" = 8
  dimension "d30" = 4.5
  constraint midpoint L1 L4.start
  constraint midpoint L3 L4.end
  constraint coincident L4 A0.centre
  measures "d29" distance of L4.start A0.centre
  measures "d30" diameter of A0
extrude "Extrude2" cut sketch "Sketch2" against normal up to surface (8.5 mm away) contours A0
sketch "Sketch3" plane through (4.25, 0, 0) normal (1, 0, 0) x (0, 0, -1)
  line L0 (-38.8384, 0) -> (-14.8384, 0)
  line L1 (-14.8384, 0) -> (-14.8384, 7.7)
  line L2 (-14.8384, 7.7) -> (-38.8384, 7.7)
  line L3 (-38.8384, 7.7) -> (-38.8384, 0)
  line L4 (-14.8384, 3.85) -> (-38.8384, 3.85) construction
  circle A0 centre (-26.8384, 3.85) radius 2.25
  line L5 (14.8384, 0) -> (26.8384, 0)
  line L6 (26.8384, 0) -> (26.8384, 7.7)
  line L7 (26.8384, 7.7) -> (14.8384, 7.7)
  line L8 (14.8384, 7.7) -> (14.8384, 0)
  line L9 (14.8384, 3.85) -> (26.8384, 3.85) construction
  circle A1 centre (20.8384, 3.85) radius 2.25
  dimension "d16" = 4.5
  constraint midpoint L1 L4.start
  constraint midpoint L3 L4.end
  constraint midpoint L4 A0.centre
  constraint midpoint L8 L9.start
  constraint midpoint L6 L9.end
  constraint midpoint L9 A1.centre
  constraint equal A0 A1
  measures "d16" diameter of A0
extrude "Extrude3" cut sketch "Sketch3" against normal up to surface (8.5 mm away) contours A0 | A1
sketch "Sketch4" plane through (0, 0, 0) normal (1, 0, 0) x (0, 0, -1)
  line L0 (-38.8384, 0) -> (-14.8384, 0) construction
  line L1 (-14.8384, 0) -> (-14.8384, 7.7) construction
  line L2 (-14.8384, 7.7) -> (-38.8384, 7.7) construction
  line L3 (-38.8384, 7.7) -> (-38.8384, 0) construction
  line L4 (14.8384, 0) -> (-14.8384, 0) construction
  line L5 (-14.8384, 0) -> (-14.8384, 7.7) construction
  line L6 (14.8384, 7.7) -> (-14.8384, 7.7) construction
  line L7 (-14.8384, 7.7) -> (-14.8384, 0) construction
  line L8 (-14.8384, 0) -> (-40.647, 0) construction
  line L9 (-40.647, 0) -> (-40.647, 7.7) construction
  line L10 (-40.647, 7.7) -> (-14.8384, 7.7) construction
  line L11 (-14.8384, 7.7) -> (-14.8384, 0) construction
  line L12 (14.8384, 0) -> (-39.7427, 0)
  line L13 (-39.7427, 0) -> (-39.7427, 7.7)
  line L14 (-39.7427, 7.7) -> (14.8384, 7.7)
  line L15 (14.8384, 7.7) -> (14.8384, 0)
  line L16 (-40.647, 7.7) -> (-38.8384, 7.7) construction
  line L17 (14.8384, 7.7) -> (14.8384, 0)
  line L18 (14.8384, 0) -> (-14.8384, 0)
  line L19 (14.8384, 0) -> (14.8384, 7.7)
  line L20 (14.8384, 7.7) -> (-14.8384, 7.7)
  circle A0 centre (20.8384, 3.85) radius 2.25
  line L21 (14.8384, 0) -> (26.8384, 0)
  line L22 (26.8384, 0) -> (26.8384, 7.7)
  line L23 (26.8384, 7.7) -> (14.8384, 7.7)
  line L24 (14.8384, 7.7) -> (14.8384, 0)
  circle A1 centre (-26.8384, 3.85) radius 2.25
  circle A2 centre (-26.8384, 3.85) radius 2.25
  constraint horizontal L12
  constraint vertical L13
  constraint horizontal L14
  constraint vertical L15
  constraint coincident L10 L13.end
  constraint coincident L4.start L12.start
  constraint coincident L9.end L10.start
  constraint coincident L2.end L3.start
  constraint midpoint L13.end L16
extrude "Extrude4" cut sketch "Sketch4" along normal blind 30 contours L12 L13 L14 L15 L17 L18 L19 L20 L24 | L15 L17 L19 L21 L22 L23 L24 | A1 A2
ref_plane "WorkPlane1" through (6.0659, 3.85, 53.3509) normal (-0.913367, 0, 0.407138) x (0.407138, 0, 0.913367)
sketch "Sketch5" plane through (-14.779, 0, 6.5878) normal (-0.913367, 0, 0.407138) x (0.407138, 0, 0.913367)
  circle A0 centre (45.204, 3.85) radius 2.25 construction
  line L0 (35.3953, 0) -> (67.0018, 0) construction
  line L1 (67.0018, 0) -> (67.0018, 7.7) construction
  line L2 (67.0018, 7.7) -> (35.3953, 7.7) construction
  line L3 (35.3953, 7.7) -> (35.3953, 0) construction
  line L4 (35.3953, 7.7) -> (51.1986, 7.7)
  line L5 (51.1986, 7.7) -> (51.1986, 0)
  line L6 (51.1986, 0) -> (35.3953, 0)
  line L7 (35.3953, 0) -> (35.3953, 7.7)
  constraint horizontal L4
  constraint vertical L5
  constraint horizontal L6
  constraint vertical L7
  constraint midpoint L0 L5.end
  constraint coincident L2.end L3.start
extrude "Extrude5" cut sketch "Sketch5" against normal up to surface (4.25 mm away)
equation "d19 = d4"
equation "d22 = d1 + 6 mm"

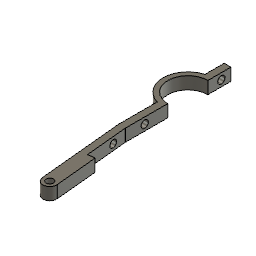
design "Trumpet Clamp 2 Main"
Autodesk Fusion 360 part; units mm, degrees
sketch "Sketch1" plane through (0, 0, 0) normal (0, 1, 0) x (1, 0, 0)
  circle A0 centre (0, 0) radius 12.435
  circle A1 centre (0, 0) radius 15.435
  line L0 (0, 0) -> (-15.435, 0) construction
  line L1 (0, 0) -> (15.435, 0) construction
  line L2 (-4.25, -39.2475) -> (0.7697, -91.2632)
  line L3 (4.25, -38.8384) -> (9.2303, -90.4468)
  circle A2 centre (5, -90.855) radius 4.25
  line L4 (5, -90.855) -> (0.7697, -91.2632) construction
  line L5 (5, -90.855) -> (9.2303, -90.4468) construction
  circle A3 centre (5, -90.855) radius 2.25
  line L6 (-4.25, -39.2475) -> (-4.25, -14.8384)
  line L7 (4.25, -38.8384) -> (4.25, -14.8384)
  line L8 (0, 0) -> (0, -38.8384) construction
  line L9 (4.25, -38.8384) -> (-4.25, -38.8384) construction
  line L10 (-4.25, 14.8384) -> (-4.25, 26.8384)
  line L11 (-4.25, 26.8384) -> (4.25, 26.8384)
  line L12 (4.25, 26.8384) -> (4.25, 14.8384)
  line L13 (-4.25, 14.8384) -> (-4.25, -14.8384) construction
  line L14 (4.25, -14.8384) -> (4.25, 14.8384) construction
  line L15 (5, -90.855) -> (5, -95.105) construction
  point P0 (0, -15.435)
  dimension "d1" = 24.87
  dimension "d3" = 4.5
  dimension "d4" = 8.5
  dimension "d5" = 5
  dimension "d19" = 8.5
  dimension "d22" = 30.87
  dimension "d27" = 24
  dimension "d28" = 12
  dimension "d32" = 79.67
  constraint coincident A0.centre A1.centre
  constraint concentric A0 A1
  constraint coincident A1 L0.end
  constraint horizontal L0
  constraint coincident A1 L1.end
  constraint parallel L0 L1
  constraint coincident A2.centre L4.start
  constraint coincident A2 L2.end
  constraint coincident A2 L3.end
  constraint parallel L4 L5
  constraint coincident L2.end L4.end
  constraint coincident L3.end L5.end
  constraint coincident A1 L6.end
  constraint coincident A1 L7.end
  constraint parallel L2 L3
  constraint vertical L6
  constraint vertical L7
  constraint vertical L8
  constraint tangent L3 A2
  constraint coincident L6 L9.end
  constraint perpendicular L6 L9
  constraint midpoint L8.end L9
  constraint coincident A1 L10.start
  constraint vertical L10
  constraint perpendicular L10 L11
  constraint coincident A1 L12.end
  constraint perpendicular L11 L12
  constraint vertical L13
  constraint vertical L14
  constraint coincident A2 L15.end
  constraint vertical L15
  constraint coincident A1 P0
  constraint coincident L8 P0
  measures "d1" diameter of A0
  measures "d3" diameter of A3
  measures "d4" diameter of A2
  measures "d5" horizontal distance of A0.centre A2.centre
  measures "d19" distance of L6 L7
  measures "d22" diameter of A1
  measures "d27" distance of L3.start L7.end
  measures "d28" distance of L11.end L12.end
  measures "d32" vertical distance of L15.end P0
extrude "Extrude1" add sketch "Sketch1" along normal blind 7.7
sketch "Sketch2" plane through (0.4974, 0, -0.048) normal (0.995376, 0, -0.096056) x (-0.096056, 0, -0.995376)
  line L0 (-90.9152, 0) -> (-39.067, 0)
  line L1 (-39.067, 0) -> (-39.067, 7.7)
  line L2 (-39.067, 7.7) -> (-90.9152, 7.7)
  line L3 (-90.9152, 7.7) -> (-90.9152, 0)
  line L4 (-39.067, 3.85) -> (-90.9152, 3.85) construction
  circle A0 centre (-47.067, 3.85) radius 2.25
  dimension "d29" = 8
  dimension "d30" = 4.5
  constraint midpoint L1 L4.start
  constraint midpoint L3 L4.end
  constraint coincident L4 A0.centre
  measures "d29" distance of L4.start A0.centre
  measures "d30" diameter of A0
extrude "Extrude2" cut sketch "Sketch2" against normal up to surface (8.5 mm away) contours A0
sketch "Sketch3" plane through (4.25, 0, 0) normal (1, 0, 0) x (0, 0, -1)
  line L0 (-38.8384, 0) -> (-14.8384, 0)
  line L1 (-14.8384, 0) -> (-14.8384, 7.7)
  line L2 (-14.8384, 7.7) -> (-38.8384, 7.7)
  line L3 (-38.8384, 7.7) -> (-38.8384, 0)
  line L4 (-14.8384, 3.85) -> (-38.8384, 3.85) construction
  circle A0 centre (-26.8384, 3.85) radius 2.25
  line L5 (14.8384, 0) -> (26.8384, 0)
  line L6 (26.8384, 0) -> (26.8384, 7.7)
  line L7 (26.8384, 7.7) -> (14.8384, 7.7)
  line L8 (14.8384, 7.7) -> (14.8384, 0)
  line L9 (14.8384, 3.85) -> (26.8384, 3.85) construction
  circle A1 centre (20.8384, 3.85) radius 2.25
  dimension "d16" = 4.5
  constraint midpoint L1 L4.start
  constraint midpoint L3 L4.end
  constraint midpoint L4 A0.centre
  constraint midpoint L8 L9.start
  constraint midpoint L6 L9.end
  constraint midpoint L9 A1.centre
  constraint equal A0 A1
  measures "d16" diameter of A0
extrude "Extrude3" cut sketch "Sketch3" against normal up to surface (8.5 mm away) contours A0 | A1
sketch "Sketch4" plane through (0, 0, 0) normal (1, 0, 0) x (0, 0, -1)
  line L0 (-38.8384, 0) -> (-14.8384, 0) construction
  line L1 (-14.8384, 0) -> (-14.8384, 7.7) construction
  line L2 (-14.8384, 7.7) -> (-38.8384, 7.7) construction
  line L3 (-38.8384, 7.7) -> (-38.8384, 0) construction
  line L4 (14.8384, 0) -> (-14.8384, 0) construction
  line L5 (-14.8384, 0) -> (-14.8384, 7.7) construction
  line L6 (14.8384, 7.7) -> (-14.8384, 7.7) construction
  line L7 (-14.8384, 7.7) -> (-14.8384, 0) construction
  line L8 (-14.8384, 0) -> (-39.2475, 0) construction
  line L9 (-39.2475, 0) -> (-39.2475, 7.7) construction
  line L10 (-39.2475, 7.7) -> (-14.8384, 7.7) construction
  line L11 (-14.8384, 7.7) -> (-14.8384, 0) construction
  line L12 (14.8384, 0) -> (-39.0429, 0)
  line L13 (-39.0429, 0) -> (-39.0429, 7.7)
  line L14 (-39.0429, 7.7) -> (14.8384, 7.7)
  line L15 (14.8384, 7.7) -> (14.8384, 0)
  line L16 (-39.2475, 7.7) -> (-38.8384, 7.7) construction
  line L17 (14.8384, 7.7) -> (14.8384, 0)
  line L18 (14.8384, 0) -> (-14.8384, 0)
  line L19 (14.8384, 0) -> (14.8384, 7.7)
  line L20 (14.8384, 7.7) -> (-14.8384, 7.7)
  circle A0 centre (20.8384, 3.85) radius 2.25
  line L21 (14.8384, 0) -> (26.8384, 0)
  line L22 (26.8384, 0) -> (26.8384, 7.7)
  line L23 (26.8384, 7.7) -> (14.8384, 7.7)
  line L24 (14.8384, 7.7) -> (14.8384, 0)
  circle A1 centre (-26.8384, 3.85) radius 2.25
  circle A2 centre (-26.8384, 3.85) radius 2.25
  constraint horizontal L12
  constraint vertical L13
  constraint horizontal L14
  constraint vertical L15
  constraint coincident L10 L13.end
  constraint coincident L4.start L12.start
  constraint coincident L9.end L10.start
  constraint coincident L2.end L3.start
  constraint midpoint L13.end L16
extrude "Extrude4" cut sketch "Sketch4" along normal blind 30 contours L12 L13 L14 L15 L17 L18 L19 L20 L24 | L15 L17 L19 L21 L22 L23 L24 | A1 A2
ref_plane "WorkPlane1" through (2.4902, 3.85, 64.8471) normal (-0.995376, 0, 0.096056) x (0.096056, 0, 0.995376)
sketch "Sketch5" plane through (-3.733, 0, 0.3602) normal (-0.995376, 0, 0.096056) x (0.096056, 0, 0.995376)
  circle A0 centre (47.067, 3.85) radius 2.25 construction
  line L0 (38.6578, 0) -> (90.9152, 0) construction
  line L1 (90.9152, 0) -> (90.9152, 7.7) construction
  line L2 (90.9152, 7.7) -> (38.6578, 7.7) construction
  line L3 (38.6578, 7.7) -> (38.6578, 0) construction
  line L4 (38.6578, 7.7) -> (64.7865, 7.7)
  line L5 (64.7865, 7.7) -> (64.7865, 0)
  line L6 (64.7865, 0) -> (38.6578, 0)
  line L7 (38.6578, 0) -> (38.6578, 7.7)
  constraint horizontal L4
  constraint vertical L5
  constraint horizontal L6
  constraint vertical L7
  constraint midpoint L0 L5.end
  constraint coincident L2.end L3.start
extrude "Extrude5" cut sketch "Sketch5" against normal up to surface (4.25 mm away)
equation "d19 = d4"
equation "d22 = d1 + 6 mm"

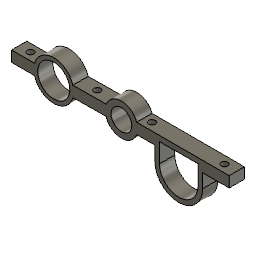
design "Trumpet Mount Far"
Autodesk Fusion 360 part; units mm, degrees
sketch "Sketch1" plane through (0, 0, 0) normal (0, 0, 1) x (1, 0, 0)
  circle A0 centre (-43.925, 0) radius 12.925
  circle A1 centre (0, 0) radius 10.5
  circle A2 centre (0, 0) radius 6.75
  line L0 (9.8995, 3.5) -> (69.8995, 3.5)
  line L1 (69.8995, 3.5) -> (69.8995, -3.5)
  line L2 (69.8995, -3.5) -> (9.8995, -3.5)
  line L3 (-31.5162, 3.6163) -> (-9.7806, 3.8197)
  line L4 (-31.4507, -3.3834) -> (-10.006, -3.1827)
  line L5 (-56.3671, 3.5) -> (-71.3671, 3.5)
  line L6 (-71.3671, 3.5) -> (-71.3671, -3.5)
  line L7 (-71.3671, -3.5) -> (-56.3671, -3.5)
  line L8 (-43.925, 0) -> (0, 0) construction
  dimension "d1" = 3.5
  dimension "d2" = 3.5
  dimension "d3" = 3.5
  dimension "d4" = 3.5
  dimension "d5" = 3.5
  dimension "d6" = 3.5
  dimension "d7" = 43.925
  dimension "d8" = 60
  dimension "d9" = 15
  dimension "d19" = 25.85
  dimension "d20" = 21
  dimension "d21" = 13.5
  constraint concentric A1 A2
  constraint coincident A1 L0.start
  constraint horizontal L0
  constraint perpendicular L0 L1
  constraint coincident A1 L2.end
  constraint perpendicular L1 L2
  constraint coincident A0 L3.start
  constraint coincident A1 L3.end
  constraint coincident A0 L4.start
  constraint coincident A1 L4.end
  constraint parallel L3 L4
  constraint coincident A0 L5.start
  constraint horizontal L5
  constraint perpendicular L5 L6
  constraint coincident A0 L7.end
  constraint perpendicular L6 L7
  constraint coincident A0.centre L8.start
  constraint coincident A1.centre A2.centre
  constraint horizontal L8
  measures "d1" distance of A1.centre L2
  measures "d2" distance of A1.centre L0
  measures "d3" distance of A0.centre L3
  measures "d4" distance of A0.centre L4
  measures "d5" distance of A0.centre L7
  measures "d6" distance of A0.centre L5
  measures "d7" horizontal distance of A0.centre A1.centre
  measures "d8" distance of L0.start L0.end
  measures "d9" distance of L5.start L5.end
  measures "d19" diameter of A0
  measures "d20" diameter of A1
  measures "d21" diameter of A2
extrude "Extrude1" add sketch "Sketch1" along normal mid plane 10